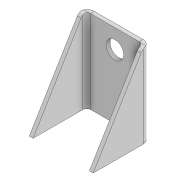
# Autodesk Inventor part: Soporte Fijo
Saved by Autodesk Inventor 2020 (Build 240168000, 168)
## iProperties
Created: 2020-03-03
Part Number: Soporte Fijo
Material: Generic
Document SubType Name: Sheet Metal
Designer: Juan Carlos Botero
Density: 1 g/cm^3
Sheet Metal Rule: Default_mm
Appearance: Default
Author: Juan Carlos Botero
Autodesk Inventor part; units mm, degrees
ref_plane "YZ Plane" through (0, 0, 0) normal (1, 0, 0) x (0, 1, 0)
ref_plane "XZ Plane" through (0, 0, 0) normal (0, 1, 0) x (-1, 0, 0)
ref_plane "XY Plane" through (0, 0, 0) normal (0, 0, 1) x (1, 0, 0)
sketch "Sketch1" plane through (0, 0, 0) normal (0, 0, 1) x (1, 0, 0)
  line L0 (-25, -32.5) -> (25, -32.5)
  line L1 (25, -32.5) -> (25, 32.5)
  line L2 (25, 32.5) -> (-25, 32.5)
  line L3 (-25, 32.5) -> (-25, -32.5)
  line L4 (-25, -32.5) -> (25, 32.5) construction
  line L5 (25, -32.5) -> (-25, 32.5) construction
  circle A0 centre (0, 17.5) radius 6.85
  point P0 (0, 0)
  dimension "d0" = 50
  dimension "d1" = 13.7
  dimension "d2" = 50
  dimension "d3" = 65
  measures "d0" distance of L0.start L0.end
  measures "d1" diameter of A0
  measures "d2" distance from line of L0 A0.centre
  measures "d3" distance of L0.end L1.end
extrude "Plate1" add sketch "Sketch1" along normal blind 3
sketch "Sketch2" plane through (-22, -32.5, 0) normal (-1, 0, 0) x (0, -1, 0)
  line L0 (-65, 0) -> (0, 0)
  line L1 (0, 0) -> (0, 45)
  line L2 (0, 45) -> (-65, 45)
  line L3 (-65, 45) -> (-65, 0)
  constraints: 6 end point, 1 horizontal, 1 perpendicular, 1 vertical
edge flange "Flange1" height 45 angle 90 thickness 3 bend radius 3 thickness toward (-1, 0, 0) relief straight relief width 3 relief depth 1.5 corner gap 3 corner form 0 edges at (-25, 0, 3) (25, 0, 3) wall of the first edge with corners at (-22, 32.5, 0) (-22, -32.5, 0) (-22, -32.5, 45) (-22, 32.5, 45)
bend "Bend1"
corner "Corner1"
sketch "Sketch3" plane through (25, -32.5, 45) normal (1, 0, 0) x (0, 0, -1)
  line L0 (0, 65) -> (0, 0) projected
  line L1 (0, 0) -> (40.9053, 68.1756)
  line L2 (40.9053, 68.1756) -> (0, 68.1756)
  line L3 (0, 68.1756) -> (0, 0)
  point P0 (45, 32.5)
  point P1 (0, 65)
  point P2 (39, 65)
  constraints: 6 end point, 2 perpendicular, 1 point on line
extrude "Extrusion1" cut sketch "Sketch3" against normal through all
fillet "Fillet1" radius 5 2 edges at (-23.5, 32.5, 6) (23.5, 32.5, 6)
equation "\"d4\" = Thickness"
equation "\"d5\" = BendReliefWidth"
equation "\"d6\" = BendReliefDepth"
equation "\"d7\" = MinimumRemnant"
equation "\"d8\" = TransitionRadius"
equation "\"d11\" = BendRadius"
equation "\"d12\" = CornerReliefSize"
equation "\"d13\" = GapSize"
equation "\"d14\" = JacobiRadiusSize"
equation "\"BendRadius\" = Thickness"
equation "\"BendReliefWidth\" = Thickness"
equation "\"BendReliefDepth\" = 0.5 * Thickness"
equation "\"CornerReliefSize\" = 4 * Thickness"
equation "\"MinimumRemnant\" = 2 * Thickness"
equation "\"TransitionRadius\" = BendRadius"
equation "\"JacobiRadiusSize\" = BendRadius"
equation "\"GapSize\" = Thickness"
equation "\"Thickness\" = 3"
body "Solid1"
